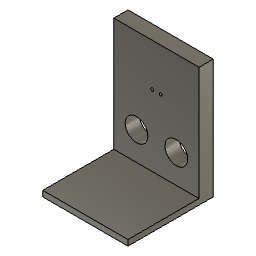
LED_Holder (Autodesk Fusion 360 design; units mm, degrees)
Autodesk Fusion 360 part; units mm, degrees
sketch "Sketch1" plane through (0, 0, 0) normal (0, 0, 1) x (1, 0, 0)
  line L0 (-15, -21) -> (15, -21)
  line L1 (15, -21) -> (15, 21)
  line L2 (15, 21) -> (-15, 21)
  line L3 (-15, 21) -> (-15, -21)
  line L4 (-15, -21) -> (15, 21) construction
  line L5 (15, -21) -> (-15, 21) construction
  line L6 (0, -21) -> (7, -21) construction
  line L7 (7, -21) -> (7, -9) construction
  line L8 (7, -9) -> (0, -9) construction
  line L9 (0, -9) -> (0, -21) construction
  line L10 (0, -21) -> (-7, -21) construction
  line L11 (-7, -21) -> (-7, -9) construction
  line L12 (-7, -9) -> (0, -9) construction
  line L13 (0, -9) -> (0, -21) construction
  circle A0 centre (-7, -9) radius 4
  circle A1 centre (7, -9) radius 4
  dimension "d1" = 30
  dimension "d2" = 42
  dimension "d3" = 7
  dimension "d4" = 12
  dimension "d5" = 7
  dimension "d6" = 12
  dimension "d7" = 8
  dimension "d8" = 8
  constraint horizontal L0
  constraint perpendicular L0 L1
  constraint parallel L0 L2
  constraint parallel L1 L3
  constraint coincident L4 origin
  constraint coincident L5 origin
  constraint horizontal L6
  constraint vertical L7
  constraint horizontal L8
  constraint vertical L9
  constraint midpoint L0 L6.start
  constraint horizontal L10
  constraint vertical L11
  constraint horizontal L12
  constraint vertical L13
  constraint coincident L11.end L12.start
  constraint coincident L7.end L8.start
  measures "d1" distance of L1.end L2.end
  measures "d2" distance of L0.end L1.end
  measures "d3" distance of L6.start L6.end
  measures "d4" distance of L6.start L8.end
  measures "d5" distance of L6.start L10.end
  measures "d6" distance of L6.start L8.end
  measures "d7" diameter of A0
  measures "d8" diameter of A1
extrude "Extrude1" add sketch "Sketch1" along normal blind 5 makes body 1
sketch "Sketch2" plane through (0, 0, 5) normal (0, 0, 1) x (-1, 0, 0)
  circle A0 centre (-7, 9) radius 4
  circle A1 centre (7, 9) radius 4
  line L0 (15, -21) -> (15, 21)
  line L1 (15, 21) -> (-15, 21)
  line L2 (-15, 21) -> (-15, -21)
  line L3 (-15, -21) -> (15, -21)
  line L4 (15, 21) -> (-15, 21)
  line L5 (-15, 21) -> (-15, 19)
  line L6 (-15, 19) -> (15, 19)
  line L7 (15, 19) -> (15, 21)
  dimension "d11" = 30
  dimension "d12" = 2
  constraint horizontal L4
  constraint vertical L5
  constraint horizontal L6
  constraint vertical L7
  constraint coincident L0.end L1.start
  measures "d11" distance of L0.end L1.end
  measures "d12" distance of L0.end L6.end
extrude "Extrude2" add sketch "Sketch2" along normal blind 25 contours L0 L1 L2 L4 L5 L6 L7 bodies 1
sketch "Sketch3" plane through (0, 0, 0) normal (0, 0, -1) x (1, 0, 0)
  circle A0 centre (7, 9) radius 4
  circle A1 centre (-7, 9) radius 4
  line L0 (-15, 21) -> (-15, -21)
  line L1 (-15, -21) -> (15, -21)
  line L2 (15, -21) -> (15, 21)
  line L3 (15, 21) -> (-15, 21)
  line L4 (0, 21) -> (-1.5, 21) construction
  line L5 (-1.5, 21) -> (-1.5, -6) construction
  line L6 (-1.5, -6) -> (0, -6) construction
  line L7 (0, -6) -> (0, 21) construction
  line L8 (0, 21) -> (1.5, 21) construction
  line L9 (1.5, 21) -> (1.5, -6) construction
  line L10 (1.5, -6) -> (0, -6) construction
  line L11 (0, -6) -> (0, 21) construction
  circle A2 centre (0, -6) radius 3.05
  circle A3 centre (-1.5, -6) radius 0.5
  circle A4 centre (1.5, -6) radius 0.5
  dimension "d15" = 1.5
  dimension "d16" = 27
  dimension "d17" = 27
  dimension "d18" = 6.1
  dimension "d19" = 1
  dimension "d20" = 1
  constraint horizontal L4
  constraint vertical L5
  constraint horizontal L6
  constraint vertical L7
  constraint midpoint L3 L4.start
  constraint horizontal L8
  constraint vertical L9
  constraint horizontal L10
  constraint vertical L11
  constraint coincident L6.end L7.start
  constraint coincident L5.end L6.start
  constraint coincident L9.end L10.start
  measures "d15" distance of L4.start L4.end
  measures "d16" distance of L4.start L6.end
  measures "d17" distance of L4.start L6.end
  measures "d18" diameter of A2
  measures "d19" diameter of A3
  measures "d20" diameter of A4
extrude "Extrude3" cut sketch "Sketch3" against normal blind 3 contours A2 bodies 1
extrude "Extrude4" cut 2 faces at (1.3037, 5.8866, 0) (-1.4875, 6.1662, 0) along direction (0, 0, -1) up to surface end surface through (0, 0, 5) normal (0, 0, 1) offset 0 on bodies 1 bodies 1
copy_body "Body->Comp1" bodies 1 removing the originals makes body 2 in component "LED_Holder"
component "LED_Holder" placed x (1, 0, 0) y (0, 1, 0) z (0, 0, 1) at (0, 0, 0)
